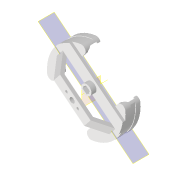
# Autodesk Inventor part: Anglerfish_Lightplate_Tosslink_flipped
Saved by Autodesk Inventor 2022 (Build 260153000, 153)
## iProperties
Created: 2022-07-21
Part Number: Anglerfish_Lightplate_Tosslink_flipped
Material: Generisch
Document SubType Name: Modeling
Designer: Muriel
Density: 1 g/cm^3
Appearance: Vorgabe
Author: Muriel
Autodesk Inventor part; units mm, degrees
ref_plane "XZ Plane" through (0, 0, 0) normal (0, 1, 0) x (-1, 0, 0)
ref_plane "XY Plane" through (0, 0, 0) normal (0, 0, 1) x (1, 0, 0)
ref_plane "Arbeitsebene4" through (0, 2.351, 3.7558) normal (1, 0, 0) x (0, 1, 0)
sketch "Skizze10" plane through (0, 2.351, 3.7558) normal (1, 0, 0) x (0, 1, 0)
  line L0 (-43.501, -12) -> (43.501, -12) projected
  line L1 (-43.501, -5.4848) -> (-43.501, -12)
  line L2 (-42.301, -11.7) -> (-42.301, -15.7)
  line L3 (-42.301, -15.7) -> (-46.301, -15.7)
  line L4 (-46.301, -15.7) -> (-46.301, 2)
  line L5 (-46.301, 2) -> (-34.301, 2)
  line L6 (-39.25, -1) -> (39.25, -1) projected
  line L7 (-34.301, 2) -> (-34.301, -1)
  line L8 (-34.301, -1) -> (-40.3733, -1)
  line L9 (-40.3733, -1) -> (-43.801, -4.4277)
  line L10 (-43.801, -4.4277) -> (-43.801, -12.3)
  line L11 (-43.801, -12.3) -> (-42.301, -11.7)
  line L12 (0, 5.54) -> (0, -19.24) projected
  line L13 (-46.301, -4.7072) -> (-45.7242, -4.7072)
  line L14 (-45.7242, -4.7072) -> (-45.7242, -9.988)
  line L15 (-45.7242, -9.988) -> (-46.301, -9.988)
  line L16 (-46.301, -9.988) -> (-46.301, -4.7072)
  point P0 (-2.351, -3.7558)
  point P1 (-42.301, -12)
  point P2 (-43.501, -11.793)
  point P3 (-43.051, -12)
  dimension "d36" = 4
  dimension "d37" = 4
  dimension "d38" = 135
  dimension "d39" = 0.3
  dimension "d40" = 2.5
  dimension "d41" = 3
  dimension "d42" = 12
  dimension "d43" = 0.6
  dimension "d56" = 0.3
  constraints: 28 end point, 5 perpendicular, 3 vertical, 2 horizontal, 2 parallel, 2 point on line, 1 other
  measures "d36" distance of L2.start L2.end
  measures "d37" distance of L2.end L3.end
  measures "d38" angle of L9 L8
  measures "d39" distance between parallel lines of L10 L1
  measures "d40" distance between parallel lines of L4 L10
  measures "d41" distance between parallel lines of L6 L5
  measures "d42" distance between parallel lines of L7 L4
  measures "d43" vertical distance of L10.end L2.start
  measures "d56" horizontal distance of L10.end L0.start
revolve "Umdrehung1" add sketch "Skizze10" angle 360 about axis through (0, 2.351, -8.2442) along (0, 0, -1) contours L0 L2 L3 L4 L15 L14 L13 L5 L7 L6 L8 L9 L10 L11
sketch "Skizze11" plane through (0, 2.351, 5.7558) normal (0, 0, 1) x (1, 0, 0)
  line L0 (-26.9619, -13.7457) -> (20.4346, 45.6645) projected
  line L1 (39.9774, 30.0736) -> (-7.4191, -29.3367) projected
  line L2 (15.5676, 59.601) -> (-54.6533, -28.4191)
  line L3 (-54.6533, -28.4191) -> (-15.5676, -59.601)
  line L4 (-15.5676, -59.601) -> (54.6533, 28.4191)
  line L5 (54.6533, 28.4191) -> (15.5676, 59.601)
  line L6 (15.5676, 59.601) -> (-15.5676, -59.601) construction
  line L7 (-54.6533, -28.4191) -> (54.6533, 28.4191) construction
  point P0 (0, -2.351)
  point P1 (0, 0)
  dimension "d45" = 50
  constraints: 12 end point, 3 parallel, 2 midpoint, 1 perpendicular
  measures "d45" distance of L3.end L2.end
extrude "Extrusion9" cut sketch "Skizze11" against normal through all
ref_plane "Arbeitsebene5" through (0, 2.351, -8.2442) normal (-0.6236376, -0.7817136, 0) x (0, 0, -1)
sketch "Skizze12" plane through (0, 2.351, -8.2442) normal (-0.6236376, -0.7817136, 0) x (0, 0, -1)
  line L0 (-14, 46.301) -> (-14, 25) projected
  line L1 (-14, -25) -> (-14, -46.301) projected
  line L2 (-14, 39.5666) -> (-30.5755, 22.9911)
  line L3 (-14, 39.5666) -> (9.4414, 39.5666) construction
  line L4 (-30.5755, 22.9911) -> (-30.5755, 0)
  line L5 (-30.5755, 0) -> (-26.5755, 0)
  line L6 (-26.5755, 0) -> (-26.5755, 21.3342)
  line L7 (-26.5755, 21.3342) -> (-14, 33.9098)
  line L8 (-14, 39.5666) -> (-14, 33.9098)
  line L9 (-38.5789, 0) -> (17.4447, 0) projected
  line L10 (-14, -46.301) -> (-14, -25)
  line L11 (-14, -39.5666) -> (-30.5755, -22.9911)
  line L12 (-30.5755, -22.9911) -> (-30.5755, 0)
  line L13 (-26.5755, 0) -> (-26.5755, -21.3342)
  line L14 (-26.5755, -21.3342) -> (-14, -33.9098)
  line L15 (-14, -39.5666) -> (-14, -33.9098)
  point P0 (-8.2442, 1.4662)
  point P1 (-8.2442, -1.4662)
  point P2 (-14, -39.5666)
  dimension "d49" = 135
  dimension "d50" = 4
  dimension "d51" = 4
  dimension "d52" = 0
  constraints: 26 end point, 5 symmetric about line, 4 point on line, 2 parallel, 2 perpendicular, 1 equal length, 1 horizontal, 1 vertical
  measures "d49" angle of L2 L3
  measures "d50" distance of L4.end L5.end
  measures "d51" distance between parallel lines of L2 L7
  measures "d52" distance between parallel lines of L5 L9
extrude "Extrusion10" add sketch "Skizze12" along normal mid plane 12
fillet "Rundung2" radius 5 8 edges at (-4.7614, -43.7045, -9.0882) (-4.7614, -43.7045, 2.4022) (-43.847, -12.5226, 2.4022) (-43.847, -12.5226, -9.0882) (43.847, 17.2247, 2.4022) (43.847, 17.2247, -9.0882) (4.7613, 48.4066, -9.0882) (4.7613, 48.4066, 2.4022)
sketch "Skizze13" plane through (0, 2.351, 5.7558) normal (0, 0, 1) x (0.9757426, -0.2189211, 0)
  arc A0 (7.4536, 6.6652) -> (0.6382, 9.9777) centre (6.3546, 13.0716) ccw projected
  arc A1 (7.4536, 6.6652) -> (0.6382, 9.9777) centre (0.0005, -0.002) ccw projected
  line L0 (10.2729, 12.2689) -> (9.4491, 10.3917) projected
  line L1 (9.4491, 10.3917) -> (9.2503, 10.479) projected
  arc A2 (9.2503, 10.479) -> (8.5915, 10.222) centre (9.0494, 10.0211) ccw projected
  line L2 (8.5915, 10.222) -> (7.9888, 8.8485) projected
  line L3 (7.9888, 8.8485) -> (2.1282, 11.4203) projected
  line L4 (2.1282, 11.4203) -> (2.7308, 12.7934) projected
  arc A3 (2.7308, 12.7934) -> (2.4729, 13.4531) centre (2.2732, 12.9948) ccw projected
  line L5 (2.4729, 13.4531) -> (2.3066, 13.5261) projected
  line L6 (2.3066, 13.5261) -> (3.1103, 15.3575) projected
  line L7 (3.1103, 15.3575) -> (3.2777, 15.2841) projected
  arc A4 (3.2777, 15.2841) -> (3.9366, 15.541) centre (3.4787, 15.7419) ccw projected
  line L8 (3.9366, 15.541) -> (4.2982, 16.3651) projected
  line L9 (4.2982, 16.3651) -> (5.6158, 16.879) projected
  line L10 (5.6158, 16.879) -> (9.6449, 15.1109) projected
  line L11 (9.6449, 15.1109) -> (10.2083, 13.7715) projected
  line L12 (10.2083, 13.7715) -> (9.8668, 12.9932) projected
  arc A5 (9.8668, 12.9932) -> (10.1237, 12.3344) centre (10.3246, 12.7923) ccw projected
  line L13 (10.1237, 12.3344) -> (10.2729, 12.2689) projected
  arc A6 (44.1629, 13.9077) -> (34.8974, 14.5927) centre (39.3938, 12.4058) ccw projected
  line L14 (34.8974, 14.5927) -> (32.7539, 10.1855) projected
  arc A7 (32.7539, -10.1855) -> (32.7539, 10.1855) centre (0, 0) ccw projected
  line L15 (32.7539, -10.1855) -> (33.1186, -9.4356) projected
  line L16 (33.1186, -9.4356) -> (38.2057, -11.9098) projected
  line L17 (38.2057, -11.9098) -> (32.9572, -22.7012) projected
  line L18 (32.9572, -22.7012) -> (27.8701, -20.227) projected
  line L19 (27.8701, -20.227) -> (28.2347, -19.4772) projected
  arc A8 (12.21, -32.0543) -> (28.2347, -19.4772) centre (0, 0) ccw projected
  line L20 (12.21, -32.0543) -> (10.0665, -36.4615) projected
  arc A9 (10.0665, -36.4615) -> (16.3259, -43.3272) centre (14.5629, -38.6484) ccw projected
  arc A10 (16.3259, -43.3272) -> (44.1629, 13.9077) centre (0, 0) ccw projected
  arc A11 (-10.0665, 36.4615) -> (-16.3259, 43.3272) centre (-14.5629, 38.6484) ccw projected
  arc A12 (-16.3259, 43.3272) -> (-44.1629, -13.9077) centre (0, 0) ccw projected
  arc A13 (-44.1629, -13.9077) -> (-34.8974, -14.5927) centre (-39.3938, -12.4058) ccw projected
  line L21 (-34.8974, -14.5927) -> (-32.7539, -10.1855) projected
  arc A14 (-32.7539, 10.1855) -> (-32.7539, -10.1855) centre (0, 0) ccw projected
  line L22 (-32.7539, 10.1855) -> (-33.1186, 9.4356) projected
  line L23 (-33.1186, 9.4356) -> (-38.2057, 11.9098) projected
  line L24 (-38.2057, 11.9098) -> (-32.9572, 22.7012) projected
  line L25 (-32.9572, 22.7012) -> (-27.8701, 20.227) projected
  line L26 (-27.8701, 20.227) -> (-28.2347, 19.4772) projected
  arc A15 (-12.21, 32.0543) -> (-28.2347, 19.4772) centre (0, 0) ccw projected
  line L27 (-12.21, 32.0543) -> (-10.0665, 36.4615) projected
  line L28 (34.8974, 14.5927) -> (32.7539, 10.1855) projected
  line L29 (32.7539, 10.1855) -> (-12.21, 32.0543)
  arc A16 (12.21, -32.0543) -> (32.7539, 10.1855) centre (0, 0) ccw projected
  line L30 (33.7499, -6.1243) -> (-25.655, 22.768)
  line L31 (-12.21, 32.0543) -> (-25.655, 38.5436)
  arc A17 (-16.3259, 43.3272) -> (-44.1629, -13.9077) centre (0, 0) ccw projected
  arc A18 (-12.21, 32.0543) -> (-28.2347, 19.4772) centre (0, 0) ccw projected
  line L32 (-25.655, 22.768) -> (-36.773, 28.1342)
  line L33 (33.7499, -6.1243) -> (44.904, -11.2878)
  arc A19 (32.7539, -10.1855) -> (32.7539, 10.1855) centre (0, 0) ccw projected
  line L34 (32.7539, 10.1855) -> (46.1371, 3.8926)
  point P0 (0.5147, -2.294)
  point P1 (9.2503, 10.479)
  point P2 (3.9366, 15.541)
  point P3 (9.8668, 12.9932)
  point P4 (10.1237, 12.3344)
  point P5 (33.7499, -6.1243)
  point P6 (-25.655, 22.768)
  point P7 (-25.655, 38.5436)
  point P8 (33.7499, -6.1243)
  constraints: 12 end point, 7 point on circle, 3 point on line, 2 parallel, 1 perpendicular
ref_plane "Arbeitsebene6" through (-40.7561, -38.405, 2.7558) normal (0, 0, 1) x (0.9992339, 0.0391365, 0)
extrude "Extrusion11" add sketch "Skizze13" along normal blind 3 contours A1 A0 | L30 A1 | A0 L30 A15 L29 A7 | A7 L34 A10 L33 | L32 A12 L31 A15
sketch "Skizze14" plane through (0, 2.351, 8.7558) normal (0, 0, 1) x (0.9757426, -0.2189211, 0)
  circle A0 centre (6.354, 13.0737) radius 6 projected
  arc A1 (7.4536, 6.6652) -> (0.6382, 9.9777) centre (6.3546, 13.0716) ccw projected
  arc A2 (7.4536, 6.6652) -> (0.6382, 9.9777) centre (0.0005, -0.002) ccw projected
  line L0 (10.2729, 12.2689) -> (9.4491, 10.3917) projected
  line L1 (9.4491, 10.3917) -> (9.2503, 10.479) projected
  arc A3 (9.2503, 10.479) -> (8.5915, 10.222) centre (9.0494, 10.0211) ccw projected
  line L2 (8.5915, 10.222) -> (7.9888, 8.8485) projected
  line L3 (7.9888, 8.8485) -> (2.1282, 11.4203) projected
  line L4 (2.1282, 11.4203) -> (2.7308, 12.7934) projected
  arc A4 (2.7308, 12.7934) -> (2.4729, 13.4531) centre (2.2732, 12.9948) ccw projected
  line L5 (2.4729, 13.4531) -> (2.3066, 13.5261) projected
  line L6 (2.3066, 13.5261) -> (3.1103, 15.3575) projected
  line L7 (3.1103, 15.3575) -> (3.2777, 15.2841) projected
  arc A5 (3.2777, 15.2841) -> (3.9366, 15.541) centre (3.4787, 15.7419) ccw projected
  line L8 (3.9366, 15.541) -> (4.2982, 16.3651) projected
  line L9 (4.2982, 16.3651) -> (5.6158, 16.879) projected
  line L10 (5.6158, 16.879) -> (9.6449, 15.1109) projected
  line L11 (9.6449, 15.1109) -> (10.2083, 13.7715) projected
  line L12 (10.2083, 13.7715) -> (9.8668, 12.9932) projected
  arc A6 (9.8668, 12.9932) -> (10.1237, 12.3344) centre (10.3246, 12.7923) ccw projected
  line L13 (10.1237, 12.3344) -> (10.2729, 12.2689) projected
  line L14 (-25.655, 22.768) -> (33.7499, -6.1243) projected
  point P0 (0.5147, -2.294)
  point P1 (1.4843, 9.5684)
  point P2 (6.6031, 7.0788)
  point P3 (9.2503, 10.479)
  point P4 (3.9366, 15.541)
  point P5 (9.8668, 12.9932)
  point P6 (10.1237, 12.3344)
extrude "Extrusion12" add sketch "Skizze14" along normal blind 6 contours A0 A2 | A2 A0 L14 picked at (3.818, 8.6873)
sketch "Skizze15" plane through (-21.7143, 11.9989, 22.3313) normal (0, 0, 1) x (0.7817136, -0.6236376, 0)
  circle A0 centre (14.4911, 6) radius 1.9 projected
  circle A1 centre (31.4911, 6) radius 1.9 projected
  circle A2 centre (22.9888, 5.9996) radius 3 projected
  circle A3 centre (14.4911, 6) radius 1.4
  circle A4 centre (31.4911, 6) radius 1.4
  point P0 (24.4573, 4.1622)
  dimension "d61" = 2.8
  dimension "d62" = 2.8
  constraints: 2 centre point, 2 coincident
  measures "d61" diameter of A3
  measures "d62" diameter of A4
extrude "Extrusion13" cut sketch "Skizze15" against normal through all contours A2 | A3 | A4
ref_plane "Arbeitsebene3" through (7.1263, -5.2789, 3.7558) normal (0, 0, 1) x (-0.6828675, 0.7305423, 0)
